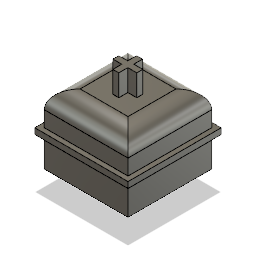
switch (Autodesk Fusion 360 design; units mm, degrees)
Autodesk Fusion 360 part; units mm, degrees
sketch "Sketch1" plane through (0, 0, 0) normal (0, 1, 0) x (1, 0, 0)
  line L0 (0, 0) -> (15.6, 0)
  line L1 (15.6, 0) -> (15.6, -15.6)
  line L2 (15.6, -15.6) -> (0, -15.6)
  line L3 (0, -15.6) -> (0, 0)
  dimension "d1" = 15.6
  dimension "d2" = 15.6
  measures "d1" distance of L0.start L0.end
  measures "d2" distance of L0.start L2.end
extrude "Extrude1" add sketch "Sketch1" along normal blind 1
sketch "Sketch4" plane through (0, 0, 0) normal (0, -1, 0) x (1, 0, 0)
  line L0 (15.6, 15.6) -> (0, 15.6)
  line L1 (0, 15.6) -> (0, 0)
  line L2 (0, 0) -> (15.6, 0)
  line L3 (15.6, 0) -> (15.6, 15.6)
  line L4 (0.8, 14.8) -> (14.8, 14.8)
  line L5 (14.8, 14.8) -> (14.8, 0.8)
  line L6 (14.8, 0.8) -> (0.8, 0.8)
  line L7 (0.8, 0.8) -> (0.8, 14.8)
  dimension "d7" = 0.8
  dimension "d8" = 0.8
  dimension "d9" = 0.8
  dimension "d10" = 0.8
  measures "d7" distance of L0 L4
  measures "d8" distance of L1 L7
  measures "d9" distance of L3 L5
  measures "d10" distance of L2 L6
extrude "Extrude2" add sketch "Sketch4" along normal blind 5 contours L4 L5 L6 L7
sketch "Sketch5" plane through (0, 1, 0) normal (0, 1, 0) x (-1, 0, 0)
  line L0 (0, 15.6) -> (-15.6, 15.6)
  line L1 (-15.6, 15.6) -> (-15.6, 0)
  line L2 (-15.6, 0) -> (0, 0)
  line L3 (0, 0) -> (0, 15.6)
  line L4 (-0.8, 0.8) -> (-14.8, 0.8)
  line L5 (-14.8, 0.8) -> (-14.8, 14.8)
  line L6 (-14.8, 14.8) -> (-0.8, 14.8)
  line L7 (-0.8, 14.8) -> (-0.8, 0.8)
  dimension "d13" = 0.8
  dimension "d14" = 0.8
  dimension "d15" = 0.8
  dimension "d16" = 0.8
  measures "d13" distance of L2 L4
  measures "d14" distance of L3 L7
  measures "d15" distance of L1 L5
  measures "d16" distance of L0 L6
extrude "Extrude3" add sketch "Sketch5" along normal blind 5.6 contours L4 L5 L6 L7
fillet "Fillet1" radius 3 4 edges at (7.8, 6.6, 0.8) (14.8, 6.6, 7.8) (7.8, 6.6, 14.8) (0.8, 6.6, 7.8)
sketch "Sketch6" plane through (0, 6.6, 0) normal (0, 1, 0) x (-1, 0, 0)
  line L0 (-3.8, 11.8) -> (-11.8, 11.8)
  line L1 (-11.8, 11.8) -> (-11.8, 3.8)
  line L2 (-11.8, 3.8) -> (-3.8, 3.8)
  line L3 (-3.8, 3.8) -> (-3.8, 11.8)
  line L4 (-8.3063, 7.3427) -> (-8.3063, 5.8427)
  line L5 (-8.3063, 7.3427) -> (-9.8063, 7.3427)
  line L6 (-8.3063, 5.8427) -> (-7.3063, 5.8427)
  line L7 (-7.3063, 5.8427) -> (-7.3063, 7.3427)
  line L8 (-7.3063, 7.3427) -> (-5.8063, 7.3427)
  line L9 (-5.8063, 7.3427) -> (-5.8063, 8.3427)
  line L10 (-5.8063, 8.3427) -> (-7.3063, 8.3427)
  line L11 (-7.3063, 8.3427) -> (-7.3063, 9.8427)
  line L12 (-7.3063, 9.8427) -> (-8.3063, 9.8427)
  line L13 (-8.3063, 9.8427) -> (-8.3063, 8.3427)
  line L14 (-8.3063, 8.3427) -> (-9.8063, 8.3427)
  line L15 (-9.8063, 8.3427) -> (-9.8063, 7.3427)
extrude "Extrude4" add sketch "Sketch6" along normal blind 3.6 contours L4 L5 L6 L7 L8 L9 L10 L11 L12 L13 L14 L15
sketch "Sketch7" plane through (0, -5, 0) normal (0, -1, 0) x (1, 0, 0)
  line L0 (0.8, 0.8) -> (14.8, 0.8)
  line L1 (14.8, 0.8) -> (14.8, 14.8)
  line L2 (14.8, 14.8) -> (0.8, 14.8)
  line L3 (0.8, 14.8) -> (0.8, 0.8)
  circle A0 centre (7.8, 7.8) radius 2.5
extrude "Extrude5" add sketch "Sketch7" along normal blind 3.3 contours A0
chamfer "Chamfer1" distance 1 angle 45 1 edges at (5.4692, -8.3, 6.896)
